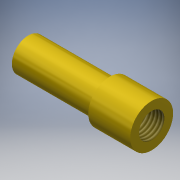
# Autodesk Inventor part: Bullet_v5_SiliconeSample_TopPart
Saved by Autodesk Inventor 2018 (Build 220112000, 112)
## iProperties
Created: 2012-08-22
Part Number: Bullet_v5_SiliconeSample_TopPart
Document SubType Name: Modeling
Designer: Sergey
Density: 8.94 g/cm^3
Material: Wrought Copper
Mass: 15.2333 g
Surface Area: 14.6745 cm^2
Volume: 1.70395 cm^3
Description: O2 free copper
Appearance: Glossy - Gold
Author: Sergey
Autodesk Inventor part; units mm, degrees
ref_plane "YZ Plane" through (0, 0, 0) normal (1, 0, 0) x (0, 1, 0)
ref_plane "XZ Plane" through (0, 0, 0) normal (0, 1, 0) x (-1, 0, 0)
ref_plane "XY Plane" through (0, 0, 0) normal (0, 0, 1) x (1, 0, 0)
sketch "Sketch1" plane through (0, 0, 0) normal (0, 0, 1) x (1, 0, 0)
  line L0 (-2.2069, 0.2356) -> (26.8656, 0.2356)
  line L1 (-2.2069, 0.2356) -> (-2.2069, 3.7916)
  line L2 (-2.2069, 3.7916) -> (8.3849, 3.7916)
  line L3 (8.3849, 3.7916) -> (9.0335, 4.8711)
  line L4 (9.0335, 4.8711) -> (21.885, 4.8711)
  line L5 (21.885, 4.8711) -> (21.885, 3.4106)
  line L6 (21.885, 3.4106) -> (23.5614, 3.4106)
  line L7 (23.5614, 3.4106) -> (23.5614, 5.5188)
  line L8 (23.5614, 5.5188) -> (31.0036, 5.5188)
  line L9 (31.0036, 5.5188) -> (31.0036, 0.2356)
  line L10 (31.0036, 0.2356) -> (-2.2069, 0.2356)
  dimension "d0" = 3.556
  dimension "d2" = 4.6355
  dimension "d3" = 121
  dimension "d5" = 25.7683
  dimension "d7" = 5.2832
  dimension "d8" = 3.175
  dimension "d56" = 15.1765
  dimension "d57" = 7.4422
  dimension "d58" = 1.6764
  dimension "d59" = 10.5918
  dimension "d60" = 33.2105
  constraints: 22 end point, 7 parallel, 2 perpendicular, 1 horizontal
  measures "d0" distance of L0.start L1.end
  measures "d2" distance between parallel lines of L4 L0
  measures "d3" angle of L3 L2
  measures "d5" distance between parallel lines of L7 L1
  measures "d7" distance between parallel lines of L8 L10
  measures "d8" distance between parallel lines of L6 L10
  measures "d56" distance from line of L2.end L7
  measures "d57" distance between parallel lines of L9 L7
  measures "d58" distance of L5.end L6.end
  measures "d59" distance of L1.end L2.end
  measures "d60" distance between parallel lines of L1 L9
revolve "Revolution1" add sketch "Sketch1" angle 360 about axis through (-2.2069, 0.2356, 0) along (1, 0, 0)
sketch "Sketch2" plane through (31.0036, 0.2356, 0) normal (1, 0, 0) x (0, 0, -1)
  circle A0 centre (0, 0) radius 5.2832 projected
  line L0 (0, 2.2914) -> (1.9844, 1.1457)
  line L1 (1.9844, 1.1457) -> (1.9844, -1.1457)
  line L2 (1.9844, -1.1457) -> (0, -2.2914)
  line L3 (0, -2.2914) -> (-1.9844, -1.1457)
  line L4 (-1.9844, -1.1457) -> (-1.9844, 1.1457)
  line L5 (-1.9844, 1.1457) -> (0, 2.2914)
  dimension "d10" = 3.9688
  constraints: 12 end point, 1 coincident, 13 other
  measures "d10" distance between parallel lines of L1 L4
extrude "Extrusion1" cut sketch "Sketch2" against normal blind 5.08 contours L0 L1 L2 L3 L4 L5
sketch "Sketch4" plane through (31.0036, 0.2356, 0) normal (1, 0, 0) x (0, 0, -1)
  circle A0 centre (0, 0) radius 5.2832 projected
  line L0 (0, 12.6958) -> (0, -10.7282) construction
  line L1 (4.6355, 2.6389) -> (4.6355, -2.6389)
  line L2 (-4.6355, 2.6389) -> (-4.6355, -2.6389)
  arc A1 (4.6355, -2.6389) -> (4.6355, 2.6389) centre (0, 0) ccw
  arc A2 (-4.6355, 2.6389) -> (-4.6355, -2.6389) centre (0, 0) ccw
  dimension "d15" = 9.271
  dimension "d16" = 4.6355
  constraints: 6 end point, 4 point on circle, 2 centre point, 2 parallel, 1 coincident
  measures "d15" distance between parallel lines of L1 L2
  measures "d16" distance from line of L1 A0.centre
sketch "Sketch7" plane through (-2.2069, 0.2356, 0) normal (-1, 0, 0) x (0, 0, 1)
  circle A0 centre (0, 0) radius 3.6195
  dimension "d53" = 7.239
  constraints: 1 centre point, 1 coincident
  measures "d53" diameter of A0
hole "Hole1" [suppressed]
sketch "Sketch9" plane through (31.0036, 0.2356, 0) normal (1, 0, 0) x (0, -1, 0)
  arc A0 (-5.2832, 0) -> (-5.2832, 0) centre (0, 0) ccw projected
  line L0 (5.7299, -0.635) -> (-5.651, -0.635)
  line L1 (-5.651, -0.635) -> (-5.651, 0.635)
  line L2 (-5.651, 0.635) -> (5.844, 0.635)
  line L3 (5.844, 0.635) -> (5.7299, -0.635)
  point P0 (0.2356, 0)
  dimension "d35" = 0.635
  dimension "d36" = 0.635
  constraints: 8 end point, 1 parallel, 1 perpendicular
  measures "d35" distance from line of L0 A0.centre
  measures "d36" distance from line of L2 A0.centre
extrude "Extrusion7" cut sketch "Sketch9" against normal blind 0.635 contours A0 L0 L2 | A0 L2 L3 L0 | A0 L0 L1 L2
sketch "Sketch10" plane through (25.9236, 0.2356, 0) normal (1, 0, 0) x (0, 0, -1)
  line L0 (0, 2.2914) -> (-1.9844, 1.1457) projected
  line L1 (-1.9844, 1.1457) -> (-1.9844, -1.1457) projected
  line L2 (-1.9844, -1.1457) -> (0, -2.2914) projected
  line L3 (0, -2.2914) -> (1.9844, -1.1457) projected
  line L4 (1.9844, -1.1457) -> (1.9844, 1.1457) projected
  line L5 (1.9844, 1.1457) -> (0, 2.2914) projected
  point P0 (0, 0)
hole "Hole2" at (25.9236, 0.2356, 0) direction (-1, 0, 0) diameter 3.2766 depth 13.97 tip angle 118
extrude "Extrusion8" cut sketch "Sketch4" against normal up to next contours A0 L1 | A0 L1 A1 | L2 A0 | A0 L2 A2
sketch "Sketch11" plane through (25.9236, 0.2356, 0) normal (1, 0, 0) x (0, 0, -1)
  circle A0 centre (0, 0) radius 1.6383 projected
  constraints: 1 coincident
hole "Hole3" at (25.9236, 0.2356, 0) direction (-1, 0, 0) diameter 1.5875 depth 31.75 tip angle 118
sketch "Sketch14" plane through (-2.2069, 0.2356, 0) normal (-1, 0, 0) x (0, 0, 1)
  circle A0 centre (0, 0) radius 0.7937 projected
  circle A1 centre (0, 0) radius 3.556 projected
  point P0 (0, -0.2356)
hole "Hole5" at (-2.2069, 0.2356, 0) direction (1, 0, 0) diameter 3.302 depth 10.3124 tip angle 118 thread size "8-32 UNC" class "2B" standard "ANSI Unified Screw Threads"
chamfer "Chamfer1" distance 0.2032 angle 59 1 edges at (25.9236, 0.2356, 1.6383) measured on face at (25.4236, 0.2356, 1.6383)
sketch "Sketch17" plane through (31.0036, -0.9101, -1.9844) normal (1, 0, 0) x (0, 0, -1)
  circle A0 centre (-1.9844, 1.1457) radius 0.7937 projected
  circle A1 centre (-1.9844, 1.1457) radius 6.6504
  point P0 (-1.9844, 0.9101)
  constraints: 1 centre point, 1 coincident
extrude "Extrusion12" cut sketch "Sketch17" against normal blind 12.9032
hole "Hole6" at (18.1004, 0.2356, 0) direction (-1, 0, 0) diameter 5.4864 depth 16.6624 tip angle 118 thread size "1/4-32 UNEF" class "2B" standard "ANSI Unified Screw Threads"
sketch "Sketch18" plane through (-2.2069, 0.2356, 0) normal (-1, 0, 0) x (0, 0, 1)
  circle A0 centre (0, 0) radius 3.556 projected
  point P0 (0, -0.2356)
extrude "Extrusion13" add sketch "Sketch18" along normal blind 6.35
ref_plane "Work Plane3" through (10.4804, 0.2356, 0) normal (1, 0, 0) x (0, 0, -1)
sketch "Sketch19" plane through (10.4804, 0.2356, 0) normal (1, 0, 0) x (0, 0, -1)
  circle A0 centre (0, 0) radius 2.7432 projected
  point P0 (0, -0.2356)
  dimension "d116" = 5.4864
  measures "d116" diameter of A0
extrude "Extrusion14" cut sketch "Sketch19" against normal blind 17.78
sketch "Sketch20" plane through (-8.5569, 0.2356, 0) normal (-1, 0, 0) x (0, 0, 1)
  circle A0 centre (0, 0) radius 3.556 projected
  point P0 (0, -0.2356)
hole "Hole7" at (-8.5569, 0.2356, 0) direction (1, 0, 0) diameter 4.064 end through all
chamfer "Chamfer2" distance 1.143 angle 45 1 edges at (-8.5569, 0.2356, -2.032)
body "Solid1"
